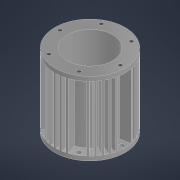
# Autodesk Inventor part: P002-Bati_chambre
Saved by Autodesk Inventor 2021.3 (Build 253353000, 353)
## iProperties
Created: 2022-03-18
Part Number: P002-Bati_chambre
Material: Aluminium
Document SubType Name: Modeling
Designer: Maintenant Prêt
Density: 2.7 g/cm^3
Appearance: Aluminum - Dark
Author: Maintenant Prêt
Autodesk Inventor part; units mm, degrees
ref_plane "YZ Plane" through (0, 0, 0) normal (1, 0, 0) x (0, 1, 0)
ref_plane "XZ Plane" through (0, 0, 0) normal (0, 1, 0) x (-1, 0, 0)
ref_plane "XY Plane" through (0, 0, 0) normal (0, 0, 1) x (1, 0, 0)
sketch "Sketch2" plane through (0, 0, 0) normal (0, 0, 1) x (1, 0, 0)
  line L0 (-25.2, 0) -> (25.2, 0) construction
  line L1 (0, -25.2) -> (0, 25.2) construction
  circle A0 centre (0, 0) radius 18
  dimension "d3" = 36
  constraints: 1 centre point, 1 coincident
  measures "d3" diameter of A0
extrude "Extrusion1" add sketch "Sketch2" along normal blind 52
sketch "Sketch3" plane through (0, 0, 52) normal (0, 0, 1) x (1, 0, 0)
  point P0 (0, 0)
hole "Hole1" at (0, 0, 52) direction (0, 0, -1) diameter 32 end through all
sketch "Sketch4" plane through (0, 0, 52) normal (0, 0, 1) x (1, 0, 0)
  circle A0 centre (0, 0) radius 20 construction
  circle A1 centre (0, 0) radius 25
  circle A2 centre (0, 0) radius 25 construction
  circle A3 centre (0, 0) radius 18
  circle A4 centre (0, 0) radius 18 construction
  constraints: 2 centre point, 2 coincident, 2 concentric
extrude "Extrusion2" add sketch "Sketch4" against normal blind 3
sketch "Sketch5" plane through (0, 0, 0) normal (0, 0, -1) x (-1, 0, 0)
  circle A0 centre (0, 0) radius 25 construction
  circle A1 centre (0, 0) radius 18 construction
  circle A2 centre (0, 0) radius 25
  circle A3 centre (0, 0) radius 18
  circle A4 centre (0, 0) radius 18 construction
  constraints: 2 centre point, 2 coincident, 2 concentric
extrude "Extrusion3" add sketch "Sketch5" against normal blind 3
sketch "Sketch6" plane through (0, 0, 52) normal (0, 0, 1) x (1, 0, 0)
  circle A0 centre (0, 0) radius 25 construction
  circle A1 centre (0, 0) radius 18 construction
  circle A2 centre (0, 0) radius 21.5 construction
  line L0 (-48.3342, 0) -> (48.3342, 0) construction
  point P0 (-21.5, 0)
  point P1 (-10.75, -18.6195)
  point P2 (10.75, -18.6195)
  point P3 (21.5, 0)
  point P4 (10.75, 18.6195)
  point P5 (-10.75, 18.6195)
  dimension "d19" = 43
  dimension "d17" = 36
  dimension "d18" = 50
  dimension "d22" = 360
  constraints: 2 end point, 1 coincident, 1 horizontal, 1 horizontal alignment, 1 point on line, 11 other
  measures "d17" diameter of A1
  measures "d18" diameter of A0
hole "Hole2" at (-21.5, 0, 52) at (-10.75, -18.6195, 52) at (10.75, -18.6195, 52) at (21.5, 0, 52) at (10.75, 18.6195, 52) at (-10.75, 18.6195, 52) direction (0, 0, -1) diameter 2.459 depth 3 thread size "M3x0.5" class "6H" standard "ISO Metric profile"
sketch "Sketch7" plane through (0, 0, 3) normal (0, 0, 1) x (1, 0, 0)
  circle A0 centre (11.25, -19.4856) radius 1.7 projected
  circle A1 centre (-22.5, 0) radius 1.7 projected
  circle A2 centre (11.25, 19.4856) radius 1.7 projected
  circle A3 centre (-11.25, 19.4856) radius 1.7 projected
  circle A4 centre (-11.25, -19.4856) radius 1.7 projected
  circle A5 centre (22.5, 0) radius 1.7 projected
  circle A6 centre (0, 0) radius 20 projected
  circle A7 centre (0, 0) radius 25 projected
hole "Hole3" at (11.25, -19.4856, 3) at (22.5, 0, 3) at (11.25, 19.4856, 3) at (-11.25, 19.4856, 3) at (-22.5, 0, 3) at (-11.25, -19.4856, 3) direction (0, 0, -1) diameter 3.4 depth 3 clearance for "Flat Head Machine Screw" size "M3" standard "Ansi Metric M Profile"
sketch "Sketch8" plane through (0, 0, 3) normal (0, 0, 1) x (1, 0, 0)
  circle A0 centre (0, 0) radius 18 construction
  circle A1 centre (0, 0) radius 18 construction
  circle A2 centre (-22.5, 0) radius 1.7 construction
  circle A3 centre (11.25, 19.4856) radius 1.7 construction
  circle A4 centre (11.25, -19.4856) radius 1.7 construction
  circle A5 centre (22.5, 0) radius 1.7 construction
  circle A6 centre (-11.25, 19.4856) radius 1.7 construction
  circle A7 centre (-11.25, -19.4856) radius 1.7 construction
  circle A8 centre (0, 0) radius 25 construction
  circle A9 centre (0, 0) radius 18 construction
  line L0 (-5.8875, -17.0099) -> (-8.177, -23.6249)
  circle A10 centre (0, 0) radius 25 construction
  line L1 (-6.8524, -24.0425) -> (-4.9338, -17.3106)
  arc A11 (-8.177, -23.6249) -> (-6.8524, -24.0425) centre (0, 0) ccw
  arc A12 (-5.8875, -17.0099) -> (-4.9338, -17.3106) centre (0, 0) ccw
  line L2 (-3.2313, -17.7076) -> (-4.488, -24.5939)
  line L3 (-3.1153, -24.8051) -> (-2.243, -17.8597)
  arc A13 (-4.488, -24.5939) -> (-3.1153, -24.8051) centre (0, 0) ccw
  arc A14 (-3.2313, -17.7076) -> (-2.243, -17.8597) centre (0, 0) ccw
  line L4 (-0.5, -17.9931) -> (-0.6944, -24.9904)
  line L5 (0.6944, -24.9904) -> (0.5, -17.9931)
  arc A15 (-0.6944, -24.9904) -> (0.6944, -24.9904) centre (0, 0) ccw
  arc A16 (-0.5, -17.9931) -> (0.5, -17.9931) centre (0, 0) ccw
  line L6 (2.243, -17.8597) -> (3.1153, -24.8051)
  line L7 (4.488, -24.5939) -> (3.2313, -17.7076)
  arc A17 (3.1153, -24.8051) -> (4.488, -24.5939) centre (0, 0) ccw
  arc A18 (2.243, -17.8597) -> (3.2313, -17.7076) centre (0, 0) ccw
  line L8 (4.9338, -17.3106) -> (6.8524, -24.0425)
  line L9 (8.177, -23.6249) -> (5.8875, -17.0099)
  arc A19 (6.8524, -24.0425) -> (8.177, -23.6249) centre (0, 0) ccw
  arc A20 (4.9338, -17.3106) -> (5.8875, -17.0099) centre (0, 0) ccw
  line L10 (-7.0323, -20.3174) -> (-11.25, -19.4856) construction
  line L11 (7.0323, -20.3174) -> (11.25, -19.4856) construction
  dimension "d39" = 1
  dimension "d42" = 35
  constraints: 24 end point, 24 point on circle, 10 centre point, 10 point on line, 7 coincident, 2 midpoint, 1 equal length, 44 other
  measures "d39" distance of L1.end L0.start
extrude "Extrusion4" add sketch "Sketch8" along normal up to surface (46 mm away)
pattern_circular "Circular Pattern1" count 6 over 360 about axis through (0, 0, -10) along (0, 0, 1) of "Extrusion4"
equation "\"d19\" = 0.5 * d18 + 0.5 * d17"
body "Solid1"
